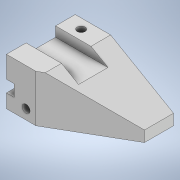
# Autodesk Inventor part: WedgeBlock
Saved by Autodesk Inventor 2022.2 (Build 262287030, 287C)
## iProperties
Created: 2023-02-22
Part Number: WedgeBlock
Material: Generic
Document SubType Name: Modeling
Designer: jak27277
Density: 1 g/cm^3
Appearance: Default
Author: jak27277
Autodesk Inventor part; units mm, degrees
ref_plane "YZ Plane" through (0, 0, 0) normal (1, 0, 0) x (0, 1, 0)
ref_plane "XZ Plane" through (0, 0, 0) normal (0, 1, 0) x (-1, 0, 0)
ref_plane "XY Plane" through (0, 0, 0) normal (0, 0, 1) x (1, 0, 0)
sketch "Sketch1" plane through (0, 0, 0) normal (1, 0, 0) x (0, 1, 0)
  line L0 (0, 0) -> (120, 0)
  line L1 (120, 0) -> (120, -175)
  line L2 (120, -175) -> (0, -175)
  line L3 (0, -175) -> (0, 0)
  dimension "d0" = 175
  dimension "d1" = 120
  constraints: 8 end point, 2 parallel, 1 horizontal, 1 perpendicular
  measures "d0" distance of L0.end L1.end
  measures "d1" distance of L0.start L0.end
extrude "Extrusion1" add sketch "Sketch1" along normal blind 250
sketch "Sketch4" plane through (250, 0, 0) normal (1, 0, 0) x (0, 0, -1)
  line L0 (175, 120) -> (0, 120) projected
  line L1 (50, 120) -> (125, 120)
  line L2 (125, 120) -> (125, 95)
  line L3 (125, 95) -> (50, 95)
  line L4 (50, 95) -> (50, 120)
  line L5 (175, 0) -> (175, 120) projected
  point P0 (0, 0)
  dimension "d6" = 75
  dimension "d7" = 50
  dimension "d8" = 25
  constraints: 8 end point, 2 parallel, 1 horizontal, 1 perpendicular, 1 point on line
  measures "d6" distance of L2.end L3.end
  measures "d7" distance between parallel lines of L5 L2
  measures "d8" distance of L3.end L1.start
extrude "Extrusion3" cut sketch "Sketch4" against normal through all
sketch "Sketch5" plane through (0, 0, 0) normal (0, 0, 1) x (1, 0, 0)
  line L0 (0, 120) -> (0, 0) projected
  line L1 (0, 35) -> (20, 35)
  line L2 (20, 35) -> (20, 65)
  line L3 (20, 65) -> (0, 65)
  line L4 (0, 65) -> (0, 35)
  circle A0 centre (50, 25) radius 10
  line L5 (0, 120) -> (250, 120) projected
  line L6 (90, 120) -> (250, 27.624)
  line L7 (250, 120) -> (250, 0) projected
  line L8 (0, 120) -> (0, 0) projected
  line L9 (0, 0) -> (250, 0) projected
  line L10 (250, 120) -> (250, 0) projected
  line L11 (0, 120) -> (250, 120) projected
  point P0 (0, 65)
  dimension "d11" = 90
  dimension "d12" = 30
  dimension "d13" = 20
  dimension "d14" = 50
  dimension "d15" = 35
  dimension "d16" = 30
  dimension "d17" = 20
  dimension "d18" = 25
  constraints: 10 end point, 3 point on line, 2 parallel, 1 centre point, 1 horizontal, 1 perpendicular
  measures "d11" distance from line of L0 L6.start
  measures "d12" angle of L5 L6
  measures "d13" diameter of A0
  measures "d14" distance from line of L0 A0.centre
  measures "d15" distance between parallel lines of L9 L1
  measures "d16" distance of L1.end L2.end
  measures "d17" distance of L2.end L3.end
  measures "d18" distance from line of L9 A0.centre
extrude "Extrusion4" cut sketch "Sketch5" against normal through all contours L3 L2 L1 L0 | L5 L7 L6 | A0
sketch "Sketch6" plane through (0, 120, -125) normal (0, 1, 0) x (1, 0, 0)
  circle A0 centre (40, 25) radius 10
  line L0 (250, 50) -> (250, -125) projected
  line L1 (250, -23.9637) -> (75, -125)
  line L2 (0, -125) -> (250, -125) projected
  line L3 (0, -75) -> (0, -125) projected
  line L4 (0, 50) -> (0, 0) projected
  line L5 (0, 50) -> (90, 50) projected
  dimension "d21" = 30
  dimension "d22" = 75
  dimension "d23" = 40
  dimension "d24" = 25
  dimension "d25" = 20
  constraints: 2 end point, 2 point on line, 1 centre point
  measures "d21" angle of L1 L2
  measures "d22" distance from line of L3 L1.end
  measures "d23" distance from line of L4 A0.centre
  measures "d24" distance from line of L5 A0.centre
  measures "d25" diameter of A0
extrude "Extrusion5" cut sketch "Sketch6" against normal through all
body "Solid1"
